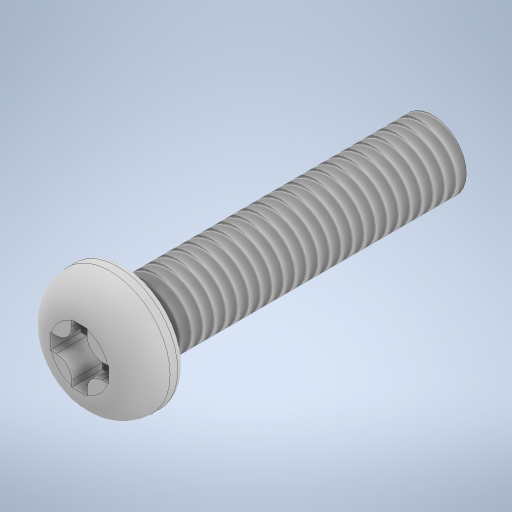
# Autodesk Inventor part: Team5_screw
Saved by Autodesk Inventor 2024 (Build 280153000, 153)
## iProperties
Created: 2024-02-23
Part Number: Team5_screw
Material: Generic
Document SubType Name: Modeling
Designer: clbri
Density: 1 g/cm^3
Appearance: Default
Author: clbri
Autodesk Inventor part; units mm, degrees
ref_plane "YZ Plane" through (0, 0, 0) normal (1, 0, 0) x (0, 1, 0)
ref_plane "XZ Plane" through (0, 0, 0) normal (0, 1, 0) x (-1, 0, 0)
ref_plane "XY Plane" through (0, 0, 0) normal (0, 0, 1) x (1, 0, 0)
sketch "Sketch1" plane through (0, 0, 0) normal (0, 0, 1) x (1, 0, 0)
  circle A0 centre (0, 0) radius 3.9
  dimension "d0" = 7.8
  constraints: 1 centre point, 1 coincident
  measures "d0" diameter of A0
extrude "Extrusion1" add sketch "Sketch1" along normal blind 3
sketch "Sketch2" plane through (0, 0, 0) normal (0, 0, -1) x (-1, 0, 0)
  circle A0 centre (0, 0) radius 2.2
  dimension "d3" = 4.4
  constraints: 1 centre point, 1 coincident
  measures "d3" diameter of A0
extrude "Extrusion2" add sketch "Sketch2" along normal blind 20
fillet "Fillet1" radius 2 1 edges at (-3.9, 0, 3)
ref_plane "Work Plane1" through (0, 0, 1) normal (0, 0, 1) x (1, 0, 0)
sketch "Sketch3" plane through (0, 0, 3) normal (0, 0, 1) x (1, 0, 0)
  line L0 (-0.5, 1.9) -> (0.5, 1.9)
  line L1 (0.5, 1.9) -> (0.5, -1.9)
  line L2 (0.5, -1.9) -> (-0.5, -1.9)
  line L3 (-0.5, -1.9) -> (-0.5, 1.9)
  line L4 (-1.9, 0.5) -> (1.9, 0.5)
  line L5 (1.9, 0.5) -> (1.9, -0.5)
  line L6 (1.9, -0.5) -> (-1.9, -0.5)
  line L7 (-1.9, -0.5) -> (-1.9, 0.5)
  point P0 (0, 0)
  point P1 (-0.5, 0.5)
  point P2 (-0.5, -0.5)
  point P3 (0.5, -0.5)
  point P4 (0.5, 0.5)
  dimension "d7" = 1
  dimension "d8" = 3.8
  dimension "d9" = 1.9
  dimension "d10" = 0.5
  dimension "d11" = 3.8
  dimension "d12" = 1
  dimension "d13" = 0.5
  dimension "d14" = 1.9
  constraints: 16 end point, 4 parallel, 2 horizontal, 2 perpendicular
  measures "d7" distance of L1.end L2.end
  measures "d8" distance of L0.end L1.end
  measures "d9" distance from line of point (0, 0) L0
  measures "d10" distance from line of point (0, 0) L3
  measures "d11" distance of L5.end L6.end
  measures "d12" distance of L4.end L5.end
  measures "d13" distance from line of point (0, 0) L4
  measures "d14" distance from line of point (0, 0) L7
extrude "Extrusion3" cut sketch "Sketch3" against normal blind 2
fillet "Fillet2" radius 1 4 edges at (-0.5, 0.5, 2) (0.5, 0.5, 2) (0.5, -0.5, 2) (-0.5, -0.5, 2)
fillet "Fillet3" radius 0.5 1 edges at (-3.9, 0, 0)
thread "Thread1" size "M4.5x0.75" class "6g" standard "ANSI Metric M Profile" length 20
body "Solid1"
